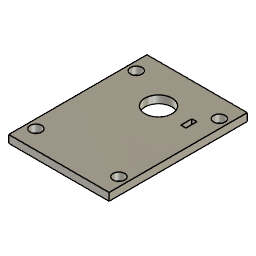
Potentiometer Case (Autodesk Fusion 360 design; units mm, degrees)
Autodesk Fusion 360 part; units mm, degrees
sketch "Sketch1" plane through (0, 0, 0) normal (0, 0, 1) x (1, 0, 0)
  line L0 (0, 0) -> (26, 0)
  line L1 (26, 0) -> (26, 35.8)
  line L2 (26, 35.8) -> (0, 35.8)
  line L3 (0, 35.8) -> (0, 0)
  circle A0 centre (23.75, 30.8) radius 1.5
  circle A1 centre (2.25, 30.8) radius 1.5
  circle A2 centre (2.25, 4.8) radius 1.5
  circle A3 centre (23.75, 4.8) radius 1.5
  circle A4 centre (13, 25.8) radius 3.5
  line L4 (21.5, 27.2) -> (20.2, 27.2)
  line L5 (20.2, 27.2) -> (20.2, 24.4)
  line L6 (20.2, 24.4) -> (21.5, 24.4)
  line L7 (21.5, 24.4) -> (21.5, 27.2)
  dimension "d1" = 26
  dimension "d2" = 35.8
  dimension "d3" = 3
  dimension "d4" = 3
  dimension "d5" = 3
  dimension "d6" = 3
  dimension "d7" = 5
  dimension "d10" = 31
  dimension "d11" = 31
  dimension "d12" = 5
  dimension "d13" = 2.25
  dimension "d14" = 2.25
  dimension "d15" = 2.25
  dimension "d16" = 2.25
  dimension "d17" = 7
  dimension "d18" = 10
  dimension "d21" = 1.3
  dimension "d22" = 2.8
  dimension "d23" = 13
  dimension "d24" = 7.2
  dimension "d25" = 8.6
  constraint horizontal L0
  constraint vertical L1
  constraint horizontal L2
  constraint vertical L3
  constraint coincident L0.start L3.end
  constraint horizontal L4
  constraint vertical L5
  constraint horizontal L6
  constraint vertical L7
  measures "d1" distance of L0.start L0.end
  measures "d2" distance of L0 L2
  measures "d3" diameter of A0
  measures "d4" diameter of A1
  measures "d5" diameter of A2
  measures "d6" diameter of A3
  measures "d7" distance of L2 A1.centre
  measures "d10" distance of L2 A2.centre
  measures "d11" distance of L2 A3.centre
  measures "d12" distance of L2 A0.centre
  measures "d13" distance of L1 A0.centre
  measures "d14" distance of L3 A1.centre
  measures "d15" distance of L3 A2.centre
  measures "d16" distance of L1 A3.centre
  measures "d17" diameter of A4
  measures "d18" distance of L2 A4.centre
  measures "d21" distance of L5 L7
  measures "d22" distance of L4 L6
  measures "d23" distance of L3 A4.centre
  measures "d24" distance of A4.centre L5
  measures "d25" distance of L2 L4
extrude "Extrude1" add sketch "Sketch1" along normal blind 2
